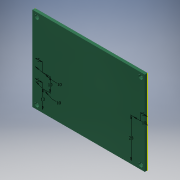
# Autodesk Inventor part: 8060모터드라이브
Saved by Autodesk Inventor 2017 (Build 210142000, 142)
## iProperties
Part Number: 8060모터드라이브
Material: 일반
Document SubType Name: Modeling
Designer: minom
Density: 1 g/cm^3
Appearance: 기본값
Author: minom
Autodesk Inventor part; units mm, degrees
ref_plane "YZ Plane" through (0, 0, 0) normal (1, 0, 0) x (0, 1, 0)
ref_plane "XZ Plane" through (0, 0, 0) normal (0, 1, 0) x (-1, 0, 0)
ref_plane "XY Plane" through (0, 0, 0) normal (0, 0, 1) x (1, 0, 0)
sketch "스케치1" plane through (0, 0, 0) normal (0, 1, 0) x (-1, 0, 0)
  line L0 (0, 0) -> (80, 0)
  line L1 (80, 0) -> (80, -60)
  line L2 (80, -60) -> (0, -60)
  line L3 (0, -60) -> (0, 0)
  dimension "d0" = 80
  dimension "d1" = 60
  constraints: 8 end point, 2 parallel, 1 horizontal, 1 perpendicular
  measures "d0" distance of L1.end L2.end
  measures "d1" distance between parallel lines of L2 L0
extrude "돌출1" add sketch "스케치1" along normal blind 2
sketch "스케치2" plane through (0, 2, 0) normal (0, 1, 0) x (1, 0, 0)
  circle A0 centre (-77, 57) radius 1.5
  circle A1 centre (-3, 57) radius 1.5
  circle A2 centre (-3, 3) radius 1.5
  circle A3 centre (-77, 3) radius 1.5
  line L0 (-80, 0) -> (-80, 60) projected
  line L1 (0, 60) -> (-80, 60) projected
  line L2 (0, 0) -> (0, 60) projected
  line L3 (-80, 0) -> (0, 0) projected
  dimension "d4" = 3
  dimension "d5" = 3
  dimension "d6" = 3
  dimension "d7" = 3
  dimension "d8" = 3
  dimension "d9" = 3
  dimension "d10" = 3
  dimension "d11" = 3
  dimension "d12" = 3
  dimension "d13" = 3
  dimension "d14" = 3
  dimension "d15" = 3
  constraints: 4 centre point
  measures "d4" diameter of A0
  measures "d5" diameter of A1
  measures "d6" diameter of A2
  measures "d7" diameter of A3
  measures "d8" distance from line of L0 A0.centre
  measures "d9" distance from line of L1 A0.centre
  measures "d10" distance from line of L2 A1.centre
  measures "d11" distance from line of L1 A1.centre
  measures "d12" distance from line of L2 A2.centre
  measures "d13" distance from line of L3 A2.centre
  measures "d14" distance from line of L3 A3.centre
  measures "d15" distance from line of L0 A3.centre
extrude "돌출2" cut sketch "스케치2" against normal blind 2 contours A0 | A1 | A2 | A3
sketch "스케치3" plane through (0, 2, 0) normal (0, 1, 0) x (1, 0, 0)
  circle A0 centre (-5, 32) radius 5
  circle A1 centre (-75, 47) radius 5
  circle A2 centre (-75, 37) radius 5
  line L0 (0, 60) -> (-80, 60) projected
  line L1 (-80, 0) -> (-80, 60) projected
  line L2 (0, 0) -> (0, 60) projected
  dimension "d18" = 10
  dimension "d19" = 10
  dimension "d20" = 10
  dimension "d21" = 10
  dimension "d22" = 13
  dimension "d23" = 5
  dimension "d24" = 5
  dimension "d25" = 5
  dimension "d26" = 28
  constraints: 3 centre point
  measures "d18" diameter of A0
  measures "d19" diameter of A1
  measures "d20" diameter of A2
  measures "d21" distance of A2.centre A1.centre
  measures "d22" distance from line of L0 A1.centre
  measures "d23" distance from line of L1 A1.centre
  measures "d24" distance from line of L1 A2.centre
  measures "d25" distance from line of L2 A0.centre
  measures "d26" distance from line of A0.centre L0
extrude "돌출3" add sketch "스케치3" along normal blind 12 contours A0 | A1 | A2
